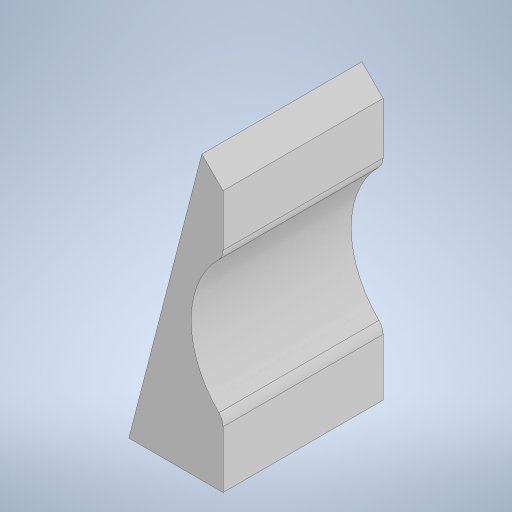
# Autodesk Inventor part: Gripper
Saved by Autodesk Inventor 2024.3 (Build 283343000, 343)
## iProperties
Created: 2025-03-19
Part Number: Gripper
Material: Generic
Document SubType Name: Modeling
Designer: migue
Density: 1 g/cm^3
Appearance: Default
Author: migue
Autodesk Inventor part; units mm, degrees
ref_plane "YZ Plane" through (0, 0, 0) normal (1, 0, 0) x (0, 1, 0)
ref_plane "XZ Plane" through (0, 0, 0) normal (0, 1, 0) x (-1, 0, 0)
ref_plane "XY Plane" through (0, 0, 0) normal (0, 0, 1) x (1, 0, 0)
sketch "Sketch1" plane through (0, 0, 0) normal (0, 1, 0) x (-1, 0, 0)
  line L0 (0, 0) -> (-20, 0)
  line L1 (-20, 0) -> (-20, -34)
  line L2 (-20, -34) -> (0, -34)
  line L3 (0, -34) -> (0, 0)
  dimension "d0" = 34
  dimension "d1" = 20
  constraints: 8 end point, 2 parallel, 1 horizontal, 1 perpendicular
  measures "d0" distance of L2.end L0.start
  measures "d1" distance of L0.start L0.end
extrude "Extrusion1" add sketch "Sketch1" along normal blind 60
chamfer "Chamfer1" distance 4.5 angle 45 1 edges at (20, 60, -17)
sketch "Sketch3" plane through (0, 0, 0) normal (0, 0, 1) x (1, 0, 0)
  line L0 (0, 60) -> (15.5, 60) projected
  line L1 (15.5, 60) -> (0, 0)
  line L2 (0, 0) -> (20, 0) projected
  line L3 (20, 0) -> (0, 0)
  line L4 (0, 0) -> (0, 60)
  line L5 (0, 60) -> (20, 60)
  line L6 (20, 60) -> (20, 0)
  constraints: 10 end point, 2 parallel, 1 horizontal, 1 perpendicular
extrude "Extrusion2" cut sketch "Sketch3" against normal blind 60 contours L0 L1 L4
sketch "Sketch4" plane through (20, 0, -34) normal (0, 0, -1) x (-1, 0, 0)
  circle A0 centre (-13.019, 28.3111) radius 19.8
  point P0 (20, 0)
  dimension "d9" = 39.6
  constraints: 1 centre point
  measures "d9" diameter of A0
extrude "Extrusion3" cut sketch "Sketch4" against normal blind 60
fillet "Fillet1" radius 3 2 edges at (20, 43.2291, -17) (20, 13.3932, -17)
shell "Shell1" thickness 1.8 removed faces 1 at (10.3333, 40, -22.6667)
body "Solid1"
